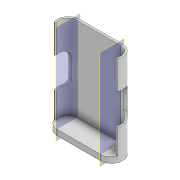
# Autodesk Inventor part: Proto-Valve Holder
Saved by Autodesk Inventor 2020 (Build 240168000, 168)
## iProperties
Created: 2019-12-04
Part Number: Proto-Valve Holder
Material: Generic
Document SubType Name: Modeling
Designer: ball
Density: 1 g/cm^3
Appearance: Default
Author: ball
Autodesk Inventor part; units mm, degrees
ref_plane "YZ Plane" through (0, 0, 0) normal (1, 0, 0) x (0, 1, 0)
ref_plane "XZ Plane" through (0, 0, 0) normal (0, 1, 0) x (-1, 0, 0)
ref_plane "XY Plane" through (0, 0, 0) normal (0, 0, 1) x (1, 0, 0)
sketch "Sketch1" plane through (0, 0, 0) normal (0, 1, 0) x (-1, 0, 0)
  line L0 (-24.3078, -12.5222) -> (24.3078, -12.5222)
  line L1 (24.3078, 12.5222) -> (-24.3078, 12.5222)
  arc A0 (24.3078, -12.5222) -> (24.3078, 12.5222) centre (24.3078, 0) ccw
  arc A1 (-24.3078, 12.5222) -> (-24.3078, -12.5222) centre (-24.3078, 0) ccw
  point P0 (0, 0)
  dimension "d2" = 25.0444
  dimension "d3" = 48.6156
  constraints: 4 end point, 4 point on circle, 4 tangent, 2 centre point, 1 horizontal, 1 parallel
  measures "d2" distance between parallel lines of L0 L1
  measures "d3" distance of A1.centre A0.centre
extrude "Extrusion1" add sketch "Sketch1" along normal blind 101.6
sketch "Sketch2" plane through (0, 101.6, 0) normal (0, 1, 0) x (1, 0, 0)
  line L0 (24.765, 10.16) -> (-24.765, 10.16)
  line L1 (-24.765, -10.16) -> (24.765, -10.16)
  arc A0 (-24.765, 10.16) -> (-24.765, -10.16) centre (-24.765, 0) ccw
  arc A1 (24.765, -10.16) -> (24.765, 10.16) centre (24.765, 0) ccw
  arc A2 (-24.3078, 12.5222) -> (-24.3078, -12.5222) centre (-24.3078, 0) ccw projected
  point P0 (0, 0)
  dimension "d7" = 20.32
  dimension "d8" = 49.53
  dimension "d16" = 0.4572
  constraints: 4 end point, 4 point on circle, 4 tangent, 2 centre point, 1 horizontal, 1 parallel
  measures "d7" distance between parallel lines of L0 L1
  measures "d8" distance of A1.centre A0.centre
  measures "d16" distance of A2.centre A0.centre
extrude "Extrusion2" cut sketch "Sketch2" against normal blind 95.25
sketch "Sketch3" plane through (0, 6.35, 0) normal (0, 1, 0) x (1, 0, 0)
  arc A0 (-24.3078, 12.5222) -> (-24.3078, -12.5222) centre (-24.3078, 0) ccw projected
  line L0 (-35.8306, -4.9022) -> (40.6958, -4.9022)
  line L1 (40.6958, -4.9022) -> (40.6958, -12.5222)
  line L2 (40.6958, -12.5222) -> (-35.8306, -12.5222)
  line L3 (-35.8306, -12.5222) -> (-35.8306, -4.9022)
  line L4 (-24.3078, -12.5222) -> (24.3078, -12.5222) projected
  point P0 (0, 0)
  dimension "d13" = 7.62
  dimension "d14" = 0
  constraints: 8 end point, 2 parallel, 1 horizontal, 1 perpendicular, 1 point on circle
  measures "d13" distance of L0.end L1.end
  measures "d14" distance between parallel lines of L2 L4
extrude "Extrusion3" cut sketch "Sketch3" along normal blind 95.25
fillet "Fillet1" radius 0.635 3 edges at (33.6641, 53.975, 4.9022) (-33.6641, 53.975, 4.9022) (-35.8306, 53.975, 4.9022)
ref_plane "Work Plane1" through (-24.765, 101.6, -10.16) normal (-1, 0, 0) x (0, -1, 0)
ref_plane "Work Plane2" through (24.765, 101.6, -10.16) normal (-1, 0, 0) x (0, -1, 0)
sketch "Sketch6" plane through (24.765, 101.6, -10.16) normal (-1, 0, 0) x (0, -1, 0)
  line L0 (66.929, 0.4433) -> (32.131, 0.4433)
  line L1 (32.131, 0.4433) -> (32.131, 26.3545)
  line L2 (32.131, 26.3545) -> (66.929, 26.3545)
  line L3 (66.929, 26.3545) -> (66.929, 0.4433)
  line L4 (95.25, 15.0622) -> (95.25, 22.6822) projected
  point P0 (101.6, 10.16)
  dimension "d30" = 34.798
  dimension "d31" = 28.321
  constraints: 8 end point, 2 parallel, 1 horizontal, 1 perpendicular
  measures "d30" distance of L1.end L2.end
  measures "d31" distance between parallel lines of L3 L4
extrude "Extrusion6" cut sketch "Sketch6" against normal up to next
fillet "Fillet3" radius 6.35 2 edges at (29.97, 34.671, -9.7167) (29.97, 69.469, -9.7167)
sketch "Sketch7" plane through (-24.765, 101.6, -10.16) normal (-1, 0, 0) x (0, -1, 0)
  line L0 (31.75, 1.1631) -> (66.04, 1.1631)
  line L1 (66.04, 1.1631) -> (66.04, 21.3162)
  line L2 (66.04, 21.3162) -> (31.75, 21.3162)
  line L3 (31.75, 21.3162) -> (31.75, 1.1631)
  line L4 (95.25, 14.6551) -> (95.25, 22.6822) projected
  point P0 (101.6, 10.16)
  dimension "d35" = 34.29
  dimension "d36" = 29.21
  constraints: 8 end point, 2 parallel, 1 horizontal, 1 perpendicular
  measures "d35" distance of L2.end L1.end
  measures "d36" distance between parallel lines of L1 L4
extrude "Extrusion7" cut sketch "Sketch7" along normal blind 25.4
fillet "Fillet4" radius 6.35 2 edges at (-31.2514, 35.56, -8.9969) (-31.2514, 69.85, -8.9969)
body "Solid1"
